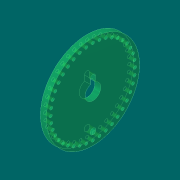
# Autodesk Inventor part: spoolBase
Saved by Autodesk Inventor 2016 (Build 200138000, 138)
## iProperties
Created: 2015-10-05
Part Number: spoolBase
Material: Polycarbonate, Clear
Document SubType Name: Modeling
Designer: Sawaiz
Density: 1.2 g/cm^3
Appearance: Clear - Green 1
Mass: 45.3403 g
Surface Area: 180.005 cm^2
Volume: 42.7739 cm^3
Author: Sawaiz
Autodesk Inventor part; units mm, degrees
ref_plane "YZ Plane" through (0, 0, 0) normal (1, 0, 0) x (0, 1, 0)
ref_plane "XZ Plane" through (0, 0, 0) normal (0, 1, 0) x (-1, 0, 0)
ref_plane "XY Plane" through (0, 0, 0) normal (0, 0, 1) x (1, 0, 0)
sketch "Sketch2" plane through (0, 0, 0) normal (1, 0, 0) x (0, 1, 0)
  circle A0 centre (0, 0) radius 47.5
  dimension "d7" = 95
  constraints: 1 centre point, 1 coincident
  measures "d7" diameter of A0
extrude "Extrusion1" add sketch "Sketch2" along normal blind 5.588
sketch "Sketch3" plane through (5.588, 0, 0) normal (1, 0, 0) x (0, 0, -1)
  circle A0 centre (0, 0) radius 47.5 projected
  line L0 (0, 0) -> (-47.5, 0)
  circle A1 centre (0, 0) radius 47.5 projected
  point P0 (-42.825, 0)
  dimension "d10" = 42.825
  constraints: 2 end point, 2 horizontal alignment, 1 horizontal, 1 point on line, 2 other
  measures "d10" distance of point (0, 0) point (-42.825, 0)
hole "Hole1" at (5.588, 0, 42.825) direction (-1, 0, 0) diameter 3.1 end through all
pattern_circular "Circular Pattern1" count 40 over 360 about axis through (-10, 0, 0) along (1, 0, 0) of "Hole1"
sketch "Sketch4" plane through (5.588, 0, 0) normal (1, 0, 0) x (0, 0, -1)
  point P0 (0, 0)
  point P1 (0, 0)
  constraints: 1 coincident
hole "Hole2" at (5.588, 0, 0) direction (-1, 0, 0) diameter 16 end through all
sketch "Sketch5" plane through (5.588, 0, 0) normal (1, 0, 0) x (0, 0, -1)
  line L0 (0, -2.5) -> (-13, -2.5)
  line L1 (-13, -2.5) -> (-13, 2.5)
  line L2 (-13, 2.5) -> (0, 2.5)
  line L3 (0, 2.5) -> (0, -2.5)
  arc A0 (-13, 2.5) -> (-13, -2.5) centre (-13, 0) ccw
  point P0 (0, 0)
  point P1 (0, 0)
  dimension "d28" = 5
  dimension "d29" = 13
  constraints: 8 end point, 2 parallel, 2 point on circle, 2 tangent, 1 centre point, 1 coincident, 1 horizontal, 1 midpoint, 1 perpendicular
  measures "d28" distance between parallel lines of L2 L0
  measures "d29" distance from line of L3 A0.centre
extrude "Extrusion2" cut sketch "Sketch5" against normal through all
sketch "Sketch6" plane through (5.588, 0, 0) normal (1, 0, 0) x (0, 0, -1)
  line L0 (-13, 2.5) -> (-7.5993, 2.5) projected
  arc A0 (-7.5993, -2.5) -> (-7.5993, 2.5) centre (0, 0) ccw projected
  line L1 (-7.5993, -2.5) -> (-13, -2.5) projected
  arc A1 (-13, 2.5) -> (-13, -2.5) centre (-13, 0) ccw projected
  circle A2 centre (-42.2978, 6.6993) radius 1.55 projected
  circle A3 centre (-40.729, 13.2337) radius 1.55 projected
  circle A4 centre (-38.1574, 19.4421) radius 1.55 projected
  circle A5 centre (-34.6462, 25.1719) radius 1.55 projected
  circle A6 centre (-30.2818, 30.2818) radius 1.55 projected
  circle A7 centre (-25.1719, 34.6462) radius 1.55 projected
  circle A8 centre (-19.4421, 38.1574) radius 1.55 projected
  circle A9 centre (-13.2337, 40.729) radius 1.55 projected
  circle A10 centre (-6.6993, 42.2978) radius 1.55 projected
  circle A11 centre (0, 42.825) radius 1.55 projected
  circle A12 centre (6.6993, 42.2978) radius 1.55 projected
  circle A13 centre (13.2337, 40.729) radius 1.55 projected
  circle A14 centre (19.4421, 38.1574) radius 1.55 projected
  circle A15 centre (25.1719, 34.6462) radius 1.55 projected
  circle A16 centre (30.2818, 30.2818) radius 1.55 projected
  circle A17 centre (34.6462, 25.1719) radius 1.55 projected
  circle A18 centre (38.1574, 19.4421) radius 1.55 projected
  circle A19 centre (40.729, 13.2337) radius 1.55 projected
  circle A20 centre (42.2978, 6.6993) radius 1.55 projected
  circle A21 centre (42.825, 0) radius 1.55 projected
  circle A22 centre (42.2978, -6.6993) radius 1.55 projected
  circle A23 centre (40.729, -13.2337) radius 1.55 projected
  circle A24 centre (38.1574, -19.4421) radius 1.55 projected
  circle A25 centre (34.6462, -25.1719) radius 1.55 projected
  circle A26 centre (30.2818, -30.2818) radius 1.55 projected
  circle A27 centre (25.1719, -34.6462) radius 1.55 projected
  circle A28 centre (19.4421, -38.1574) radius 1.55 projected
  circle A29 centre (13.2337, -40.729) radius 1.55 projected
  circle A30 centre (6.6993, -42.2978) radius 1.55 projected
  circle A31 centre (0, -42.825) radius 1.55 projected
  circle A32 centre (-6.6993, -42.2978) radius 1.55 projected
  circle A33 centre (-13.2337, -40.729) radius 1.55 projected
  circle A34 centre (-19.4421, -38.1574) radius 1.55 projected
  circle A35 centre (-25.1719, -34.6462) radius 1.55 projected
  circle A36 centre (-30.2818, -30.2818) radius 1.55 projected
  circle A37 centre (-34.6462, -25.1719) radius 1.55 projected
  circle A38 centre (-38.1574, -19.4421) radius 1.55 projected
  circle A39 centre (-40.729, -13.2337) radius 1.55 projected
  circle A40 centre (-42.2978, -6.6993) radius 1.55 projected
  circle A41 centre (-42.825, 0) radius 1.55 projected
  circle A42 centre (0, 0) radius 47.5 projected
  point P0 (34.825, 0)
  dimension "d32" = 8
  dimension "d33" = 0
  measures "d32" distance of point (34.825, 0) A21.centre
  measures "d33" vertical distance of A21.centre point (34.825, 0)
hole "Hole3" at (5.588, 0, -34.825) direction (-1, 0, 0) diameter 6 end through all
equation "\"d7\" = spoolDiameter"
equation "\"d8\" = spoolThickness"
equation "\"d10\" = -0.5 * cardPinDiameter + 0.5 * spoolDiameter - materialThickness"
equation "\"d34\" = magnetDiameter"
equation "\"materialThickness\" = 3.175"
equation "\"laserKerf\" = 0.1"
equation "\"cardPinDiameter\" = 3"
equation "\"spoolDiameter\" = 95"
equation "\"centeralShaftDiameter\" = 8"
equation "\"cardHeight\" = 53.98"
equation "\"cardWidth\" = 85.6"
equation "\"cardThickness\" = 0.76"
equation "\"cardFillet\" = 2.88"
equation "\"cardClearence\" = 0.5"
equation "\"bearingOd\" = 22"
equation "\"bearingWidth\" = 8"
equation "\"axleHeight\" = 95"
equation "\"nutTrapDepth\" = 2.5"
equation "\"nutTrapwidth\" = 5.5"
equation "\"nutTrapClearence\" = 2"
equation "\"magnetLength\" = 3"
equation "\"magnetDiameter\" = 6"
equation "\"magnetProtusion\" = 0.25"
equation "\"spoolThickness\" = 5.588"
body "Solid1"
